Autodesk Fusion 360 part; units mm, degrees
note: some values were not read from the file. Set by a fixed rule: which sketch regions a step uses.
(part 6 of 6)
  measures "d73" distance of A156.centre A157.centre
  measures "d74" distance of A156.centre A158.centre
  measures "d75" diameter of A156
  measures "d76" diameter of A157
  measures "d77" diameter of A158
  measures "d78" diameter of A159
  measures "d86" distance of L4220.start L4220.end
  measures "d87" distance of L4220.start L4222.end
  measures "d96" distance of L4224.start L4224.end
  measures "d97" distance of L4224.start L4226.end
  measures "d98" distance of L4228.start L4228.end
  measures "d99" distance of L4228.start L4230.end
  measures "d100" diameter of A160
  measures "d114" distance of L4252.end L4258.start
  measures "d115" distance of L4252.end L4252.start
  measures "d116" distance of L4264.start L4266.start
  measures "d117" distance of L4254.end L4266.start
  measures "d118" distance of L4253.end L4273.end
  measures "d119" distance of L4253.end L4253.start
  measures "d120" distance of L4257.start L4257.end
  measures "d121" distance of L4257.start L4248.end
  measures "d122" distance of L4249.start L4249.end
  measures "d123" distance of L4249.start L4267.end
  measures "d124" distance of L4250.start L4259.start
  measures "d125" distance of L4259.start L4247.end
  measures "d126" diameter of A161
  measures "d127" distance of L4256.start L4261.start
  measures "d128" distance of L4251 L4254
  measures "d129" distance of L4251 L4261
  measures "d131" diameter of A162
  measures "d134" diameter of A163
  measures "d137" diameter of A164
  measures "d140" diameter of A165
  measures "d149" diameter of A166
  measures "d152" diameter of A167
  measures "d153" diameter of A168
  measures "d154" diameter of A169
  measures "d161" distance of L4232 L4245
  measures "d168" diameter of A170
  measures "d169" diameter of A171
  measures "d170" diameter of A172
  measures "d171" diameter of A173
  measures "d212" distance of L4303.end L4304.end
  measures "d221" distance of L4315.start L4315.end
  measures "d222" distance of L4315.start L4317.end
  measures "d226" distance of L4319.start L4319.end
  measures "d227" distance of L4319.start L4321.end
  measures "d238" distance of L4312 L4313
  measures "d241" distance of L132 L4309
extrude "Extrude1" add sketch "300mm" along normal blind 3 contours L284 L285 L286 L287 L288 L289 L290 L291 L292 L293 L294 L295 L296 L297 L298 L299 L300 L301 L302 L303 L304 L305 L306 L307 L308 L309 L310 L311 L312 L313 L314 L315 L316 L317 L318 L319 L320 L321 L322 L323 L324 L325 L326 L327 L328 L329 L330 L331 L332 L333 L334 L335 L336 L337 L338 L339 L340 L341 L342 L343 L344 L345 L346 L347 L348 L349 L350 L351 L352 L353 L354 L355 | L4216 A144 L4217 A145 L4218 A146 L4219 A151 makes body 1
extrude "Extrude10" add sketch "300mm" along normal blind 3 separate body contours L0 L1 L2 L3 L4 L5 L6 L7 L8 L9 L10 L11 L12 L13 L14 L15 L16 L17 L18 L19 L20 L21 L22 L23 L24 L25 L26 L27 L28 L29 L30 L31 L32 L33 L34 L35 L36 L37 L38 L39 L40 L41 L42 L43 L44 L45 L46 L47 L48 L49 L50 L51 L52 L53 L54 L55 L56 L57 L58 L59 L60 L61 L62 L63 L64 L65 L66 L67 L68 L69 L70 L71 L72 L73 L74 L75 L76 L77 makes body 2
move_body "Move5" bodies 2 to x (1, 0, 0) y (0, 0, 1) z (0, -1, 0) at (0, 6, 0)
move_body "Align3" bodies 2 to x (1, 0, 0) y (0, 1, 0) z (0, 0, 1) at (444, 135, -3)
extrude "Extrude12" add sketch "300mm" along normal blind 3 separate body contours L4232 L4233 L4234 L4235 L4236 L4237 L4238 L4239 L4240 L4241 L4242 L4243 L4244 L4245 L4246 makes body 3
extrude "Extrude13" add sketch "300mm" along normal blind 3 separate body contours L4283 L4284 L4285 L4286 L4287 L4288 L4289 L4290 L4291 L4292 L4293 L4294 L4295 L4296 L4297 L4303 L4304 L4305 L4306 makes body 4
move_body "Move7" bodies 4 to x (1, 0, 0) y (0, 1, 0) z (0, 0, 1) at (0, 285, 174)
move_body "Move8" bodies 3 to x (1, 0, 0) y (0, 1, 0) z (0, 0, 1) at (-309.5, 135, 138)
move_body "Move9" bodies 4 to x (1, 0, 0) y (0, 1, 0) z (0, 0, 1) at (0, 0, 50)
move_body "Move10" bodies 3 to x (1, 0, 0) y (0, 0.547826, 0.836592) z (0, -0.836592, 0.547826) at (0, 122.4812, 55.3906)
move_body "Move11" bodies 4 to x (1, 0, 0) y (0, 1, 0) z (0, 0, 1) at (0, 0, 11.1)
move_body "Align6" bodies 3 to x (1, 0, 0) y (0, 1, 0) z (0, 0, 1) at (308.3, 128.4902, -1.3565)
move_body "Move12" bodies 4 to x (1, 0, 0) y (0, 1, 0) z (0, 0, 1) at (0, 0, -1)
extrude "Extrude17" add sketch "300mm" along normal blind 3 separate body contours L160 L161 L162 L163 L164 L165 L166 L167 L168 L169 L170 L171 L172 L173 L174 L175 L176 L177 L178 L179 L180 L181 L182 L183 L184 L185 L186 L187 L188 L189 L190 L191 L192 L193 L194 L195 L196 L197 L198 L199 L200 L201 L202 L203 L204 L205 L206 L207 L208 L209 L210 L211 L212 L213 L214 L215 L216 L217 L218 L219 L220 L221 L222 L223 L224 L225 L226 L227 L228 L229 L230 L231 L232 L233 L234 L235 L236 L237 L4300 L4301 makes body 5
move_body "Move15" bodies 5 to x (1, 0, 0) y (0, 0, 1) z (0, -1, 0) at (0, 150, -144)
move_body "Align10" bodies 5 to x (1, 0, 0) y (0, 1, 0) z (0, 0, 1) at (444, 120, -3)
extrude "Extrude18" add sketch "300mm" along normal blind 3 separate body contours L118 L119 L120 L121 L122 L123 L124 L125 L126 L127 L128 L129 L130 L131 L132 L133 L134 L135 L136 L137 L138 L139 L140 L141 L142 L143 L144 L145 L146 L147 L148 L149 L150 L151 L152 L153 L154 L155 L156 L157 L158 L159 L4298 L4299 L4309 L4310 L4311 makes body 6
move_body "Align11" bodies 6 to x (1, 0, 0) y (0, 1, 0) z (0, 0, 1) at (0, 135, 138)
extrude "Extrude19" add sketch "300mm" along normal blind 3 separate body contours L238 L239 L240 L241 L242 L243 L244 L245 L246 L247 L248 L249 L250 L251 L252 L253 L254 L255 L256 L257 L258 L259 L260 L261 L262 L263 L264 L265 L266 L267 L268 L269 L270 L271 L272 L273 L274 L275 L276 L277 L278 L279 L280 L281 L282 L283 makes body 7
move_body "Move16" bodies 7 to x (1, 0, 0) y (0, 0, 1) z (0, -1, 0) at (0, 150, -144)
move_body "Move17" bodies 7 to x (0, -1, 0) y (1, 0, 0) z (0, 0, 1) at (159, 459, 0)
move_body "Align12" bodies 7 to x (1, 0, 0) y (0, 1, 0) z (0, 0, 1) at (138, 120, -3)
extrude "Extrude20" add sketch "300mm" along normal blind 3 separate body contours L78 L79 L80 L81 L82 L83 L84 L85 L86 L87 L88 L89 L90 L91 L92 L93 L94 L95 L96 L97 L98 L99 L100 L101 L102 L103 L104 L105 L106 L107 L108 L109 L110 L111 L112 L113 L114 L115 L116 L117 L4302 L4307 L4308 makes body 8
move_body "Move18" bodies 8 to x (1, 0, 0) y (0, 0, 1) z (0, -1, 0) at (0, -144, 150)
move_body "Move19" bodies 8 to x (0, 1, 0) y (-1, 0, 0) z (0, 0, 1) at (165, -459, 0)
move_body "Align13" bodies 8 to x (1, 0, 0) y (0, 1, 0) z (0, 0, 1) at (269.2, 293, -3.047)
move_body "Align14" bodies 4 to x (1, 0, 0) y (0, 1, 0) z (0, 0, 1) at (168.8, -5, 0.047)
move_body "Align15" bodies 8 to x (1, 0, 0) y (0, 1, 0) z (0, 0, 1) at (168.8, -5, 0.047)
extrude "Extrude6" [rolled back] along distance 3 taper angle 0
extrude "Extrude7" [rolled back] along distance 3 taper angle 0
extrude "Extrude4" [rolled back] along distance 3 taper angle 0
extrude "Extrude5" [rolled back] along distance 3 taper angle 0
extrude "Extrude2" [rolled back] along distance 3 taper angle 0
extrude "Extrude3" [rolled back] along distance 3 taper angle 0
named bodies: "Bottom", "Left", "Right", "Front", "Control", "NFC", "Rear", "Top"
